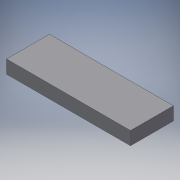
# Autodesk Inventor part: APOIO_PERFIL_STRUTURAL
Saved by Autodesk Inventor 2018 (Build 220112000, 112)
## iProperties
Created: 2018-10-09
Part Number: APOIO_PERFIL_STRUTURAL
Material: Genérico
Document SubType Name: Modeling
Designer: Georgines
Density: 1 g/cm^3
Appearance: Padrão
Author: Georgines
Autodesk Inventor part; units mm, degrees
ref_plane "YZ Plane" through (0, 0, 0) normal (1, 0, 0) x (0, 1, 0)
ref_plane "XZ Plane" through (0, 0, 0) normal (0, 1, 0) x (-1, 0, 0)
ref_plane "XY Plane" through (0, 0, 0) normal (0, 0, 1) x (1, 0, 0)
sketch "Esboço1" plane through (0, 0, 0) normal (0, 0, 1) x (1, 0, 0)
  line L0 (25, 21.6235) -> (-105, 21.6235)
  line L1 (-105, 21.6235) -> (-105, 66.6235)
  line L2 (-105, 66.6235) -> (25, 66.6235)
  line L3 (25, 66.6235) -> (25, 21.6235)
  dimension "d13" = 130
  dimension "d14" = 45
  constraints: 8 end point, 2 parallel, 1 horizontal, 1 perpendicular
  measures "d13" distance of L0.start L0.end
  measures "d14" distance of L0.end L1.end
extrude "Extrusão1" add sketch "Esboço1" along normal blind 13.8545
